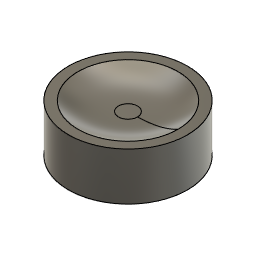
JoyPad v4 (Autodesk Fusion 360 design; units mm, degrees)
Autodesk Fusion 360 part; units mm, degrees
sketch "スケッチ1" plane through (0, 0, 0) normal (0, 0, 1) x (1, 0, 0)
  line L0 (0, 0) -> (0.238, 0)
  line L1 (0.238, 0) -> (6.238, 0)
  line L2 (6.238, 0) -> (6.238, 4)
  line L3 (0, 0) -> (0, 3)
  line L4 (0, 3) -> (1, 3)
  line L5 (6.238, 4) -> (5.238, 4)
  spline S0 degree 5 poles (1, 3) (1.1004, 3.0037) (1.2998, 3.0125) (1.5949, 3.0299) (1.9802, 3.0617) (2.4472, 3.1166) (2.8983, 3.1882) (3.3319, 3.2779) (3.7472, 3.3868) (4.1446, 3.5143) (4.5253, 3.6593) (4.8176, 3.7881) (5.0303, 3.8915) (5.1692, 3.9633) (5.238, 4) knots 0 0 0 0 0 0 0.1 0.2 0.3 0.4 0.5 0.6 0.7 0.8 0.9 1 1 1 1 1 1
  point P0 (3.4, 3.3)
  dimension "d1" = 6
  dimension "d2" = 4
  dimension "d3" = 3
  dimension "d4" = 1
  constraint coincident L0.start L3.start
  constraint horizontal L0
  constraint parallel L0 L1
  constraint perpendicular L1 L2
  constraint perpendicular L0 L3
  constraint perpendicular L3 L4
  constraint perpendicular L2 L5
  measures "d1" distance of L0.end L1.end
  measures "d2" distance of L1.end L2.end
  measures "d3" distance of L0.start L3.end
  measures "d4" distance of L2.end L5.end
revolve "回転1" add sketch "スケッチ1" angle 360 about axis through (0, 0, 0) along (0, 1, 0)
sketch "スケッチ2" plane through (0, 0, 0) normal (0, -1, 0) x (1, 0, 0)
  circle A0 centre (0, 0) radius 6.238
  circle A1 centre (0, 0) radius 2.1
  line L0 (0, 0) -> (0, 1.5)
  line L1 (0, 1.5) -> (1.4697, 1.5)
  line L2 (0, 1.5) -> (-1.4697, 1.5)
  line L3 (0, 0) -> (0, -1.5)
  line L4 (0, -1.5) -> (1.4697, -1.5)
  line L5 (0, -1.5) -> (-1.4697, -1.5)
  dimension "d6" = 4.2
  dimension "d7" = 1.5
  dimension "d8" = 1.5
  constraint coincident A0.centre A1.centre
  constraint vertical L0
  constraint coincident A1 L1.end
  constraint perpendicular L0 L1
  constraint coincident A1 L2.end
  constraint perpendicular L0 L2
  constraint parallel L0 L3
  constraint coincident A1 L4.end
  constraint perpendicular L3 L4
  constraint coincident A1 L5.end
  constraint perpendicular L3 L5
  measures "d6" diameter of A1
  measures "d7" distance of A0.centre L0.end
  measures "d8" distance of A0.centre L3.end
extrude "押し出し1" cut sketch "スケッチ2" against normal blind 2 contours A1 L0 L1 L3 L4 | A1 L0 L2 L3 L5
sketch "スケッチ3" plane through (0, 0, 0) normal (0, -1, 0) x (1, 0, 0)
  line L0 (-1.4697, 1.5) -> (1.4697, 1.5)
  arc A0 (1.4697, -1.5) -> (1.4697, 1.5) centre (0, 0) ccw
  line L1 (1.4697, -1.5) -> (-1.4697, -1.5)
  arc A1 (-1.4697, 1.5) -> (-1.4697, -1.5) centre (0, 0) ccw
  circle A2 centre (0, 0) radius 6.238
  line L2 (0, 1.5) -> (0.2, 1.5)
  line L3 (0, 1.5) -> (-0.2, 1.5)
  line L4 (0, 1.5) -> (0, 1.7)
  line L5 (-0.2, 1.5) -> (0, 1.7)
  line L6 (0, 1.7) -> (0.2, 1.5)
  line L7 (0, -1.5) -> (0.2, -1.5)
  line L8 (0, -1.5) -> (-0.2, -1.5)
  line L9 (0, -1.5) -> (0, -1.7)
  line L10 (0, -1.7) -> (0.2, -1.5)
  line L11 (-0.2, -1.5) -> (0, -1.7)
  dimension "d11" = 0.2
  dimension "d12" = 0.2
  dimension "d13" = 0.2
  dimension "d14" = 0.2
  dimension "d15" = 0.2
  dimension "d16" = 0.2
  constraint midpoint L0 L2.start
  constraint parallel L0 L2
  constraint parallel L0 L3
  constraint perpendicular L2 L4
  constraint midpoint L1 L7.start
  constraint parallel L1 L7
  constraint parallel L1 L8
  constraint perpendicular L8 L9
  measures "d11" distance of L2.start L2.end
  measures "d12" distance of L2.start L3.end
  measures "d13" distance of L2.start L4.end
  measures "d14" distance of L7.start L7.end
  measures "d15" distance of L7.start L8.end
  measures "d16" distance of L7.start L9.end
extrude "押し出し2" cut sketch "スケッチ3" against normal blind 2 contours L0 L3 L4 L5 | L0 L2 L4 L6 | L1 L8 L9 L11 | L1 L7 L9 L10
sketch "スケッチ4" plane through (0, 0, 0) normal (0, -1, 0) x (1, 0, 0)
  line L0 (0, 1.7) -> (0.2, 1.5)
  line L1 (0.2, 1.5) -> (1.4697, 1.5)
  arc A0 (1.4697, -1.5) -> (1.4697, 1.5) centre (0, 0) ccw
  line L2 (1.4697, -1.5) -> (0.2, -1.5)
  line L3 (0.2, -1.5) -> (0, -1.7)
  line L4 (0, -1.7) -> (-0.2, -1.5)
  line L5 (-0.2, -1.5) -> (-1.4697, -1.5)
  arc A1 (-1.4697, 1.5) -> (-1.4697, -1.5) centre (0, 0) ccw
  line L6 (-1.4697, 1.5) -> (-0.2, 1.5)
  line L7 (-0.2, 1.5) -> (0, 1.7)
  circle A2 centre (0, 0) radius 6.238
  line L8 (0, 1.5586) -> (0.1586, 1.4)
  line L9 (0.1586, 1.4) -> (1.4283, 1.4)
  arc A3 (1.4283, -1.4) -> (1.4283, 1.4) centre (0, 0) ccw
  line L10 (1.4283, -1.4) -> (0.1586, -1.4)
  line L11 (0.1586, -1.4) -> (0, -1.5586)
  line L12 (0, -1.5586) -> (-0.1586, -1.4)
  line L13 (-0.1586, -1.4) -> (-1.4283, -1.4)
  arc A4 (-1.4283, 1.4) -> (-1.4283, -1.4) centre (0, 0) ccw
  line L14 (-1.4283, 1.4) -> (-0.1586, 1.4)
  line L15 (-0.1586, 1.4) -> (0, 1.5586)
  dimension "d19" = 0.1
extrude "押し出し3" add sketch "スケッチ4" against normal blind 2 contours L0 L1 A0 L2 L3 L4 L5 A1 L6 L7
extrude "押し出し4" add 1 faces at (0.9388, 0, -3.0134) along direction (0, -1, 0) blind 1
sketch "スケッチ5" plane through (0, -1, 0) normal (0, -1, 0) x (1, 0, 0)
  arc A0 (-1.4283, 1.4) -> (-1.4283, -1.4) centre (0, 0) ccw
  line L0 (-1.4283, 1.4) -> (-0.1586, 1.4)
  line L1 (-0.1586, 1.4) -> (0, 1.5586)
  line L2 (0, 1.5586) -> (0.1586, 1.4)
  line L3 (0.1586, 1.4) -> (1.4283, 1.4)
  arc A1 (1.4283, -1.4) -> (1.4283, 1.4) centre (0, 0) ccw
  line L4 (1.4283, -1.4) -> (0.1586, -1.4)
  line L5 (0.1586, -1.4) -> (0, -1.5586)
  line L6 (0, -1.5586) -> (-0.1586, -1.4)
  line L7 (-0.1586, -1.4) -> (-1.4283, -1.4)
  circle A2 centre (0, 0) radius 6.238
  line L8 (0, 1.7) -> (0.2, 1.5)
  line L9 (0.2, 1.5) -> (1.4697, 1.5)
  arc A3 (1.4697, -1.5) -> (1.4697, 1.5) centre (0, 0) ccw
  line L10 (1.4697, -1.5) -> (0.2, -1.5)
  line L11 (0.2, -1.5) -> (0, -1.7)
  line L12 (0, -1.7) -> (-0.2, -1.5)
  line L13 (-0.2, -1.5) -> (-1.4697, -1.5)
  arc A4 (-1.4697, 1.5) -> (-1.4697, -1.5) centre (0, 0) ccw
  line L14 (-1.4697, 1.5) -> (-0.2, 1.5)
  line L15 (-0.2, 1.5) -> (0, 1.7)
  dimension "d24" = -0.1
extrude "押し出し5" cut sketch "スケッチ5" against normal blind 3 contours L8 L9 A3 L10 L11 L12 L13 A4 L14 L15
sketch "スケッチ6" plane through (0, -1, 0) normal (0, -1, 0) x (1, 0, 0)
  line L0 (-0.2, -1.5) -> (-1.4697, -1.5)
  arc A0 (-1.4697, 1.5) -> (-1.4697, -1.5) centre (0, 0) ccw
  line L1 (-1.4697, 1.5) -> (-0.2, 1.5)
  line L2 (-0.2, 1.5) -> (0, 1.7)
  line L3 (0, 1.7) -> (0.2, 1.5)
  line L4 (0.2, 1.5) -> (1.4697, 1.5)
  arc A1 (1.4697, -1.5) -> (1.4697, 1.5) centre (0, 0) ccw
  line L5 (1.4697, -1.5) -> (0.2, -1.5)
  line L6 (0.2, -1.5) -> (0, -1.7)
  line L7 (0, -1.7) -> (-0.2, -1.5)
  circle A2 centre (0, 0) radius 6.238
  line L8 (-0.1793, -1.45) -> (-1.4491, -1.45)
  arc A3 (-1.4491, 1.45) -> (-1.4491, -1.45) centre (0, 0) ccw
  line L9 (-1.4491, 1.45) -> (-0.1793, 1.45)
  line L10 (-0.1793, 1.45) -> (0, 1.6293)
  line L11 (0, 1.6293) -> (0.1793, 1.45)
  line L12 (0.1793, 1.45) -> (1.4491, 1.45)
  arc A4 (1.4491, -1.45) -> (1.4491, 1.45) centre (0, 0) ccw
  line L13 (1.4491, -1.45) -> (0.1793, -1.45)
  line L14 (0.1793, -1.45) -> (0, -1.6293)
  line L15 (0, -1.6293) -> (-0.1793, -1.45)
  line L16 (-1.4491, 1.45) -> (-1.3991, 1.5)
  line L17 (-1.4491, -1.45) -> (-1.3991, -1.5)
  line L18 (1.4491, -1.45) -> (1.3991, -1.5)
  line L19 (1.4491, 1.45) -> (1.3991, 1.5)
  dimension "d27" = -0.05
  constraint coincident L1 L16.end
  constraint tangent A3 L16
  constraint coincident L0 L17.end
  constraint tangent A3 L17
  constraint coincident L5 L18.end
  constraint tangent A4 L18
  constraint coincident L4 L19.end
  constraint tangent A4 L19
extrude "押し出し6" add sketch "スケッチ6" against normal blind 3 contours L0 A0 L1 A3 L16 L17 | L4 A1 L5 A4 L18 L19
